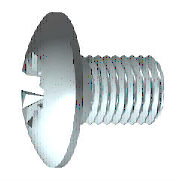
# Autodesk Inventor part: ANSI B18.6.3 - No. 2 - 56 - 5/8, CRTHMSTII(1)
Saved by Autodesk Inventor 2022.3 (Build 263350000, 350)
## iProperties
Created: 2021-02-01
Part Number: ANSI B18.6.3 - No. 2 - 56 - 5/8, CRTHMSTII(1)
Material: Steel, Mild
Description: Cross Recessed Truss Head Machine Screw - Type IA
Document SubType Name: Modeling
Standard: ANSI B18.6.3
Designer: Nathan Cai
Standard Revision: 2003
Standards Organization: ANSI
Language: en-US
Size Designation: No. 2 - 56 - 5/8
Categories: <MemberInstance><Categories><Category DisplayName="Fasteners" InternalName="e4da775c-781d-43d5-af7c-5136215cf5a6" Mnemonic="FSTN"><Category DisplayName="Bolts" InternalName="536e6df0-f778-49ac-b2f2-25c71d2aa0b2" Mnemonic="SCRW"><CategoryParameter DisplayName="Nominal Diameter Designation" InternalName="03caf894-eafd-4c09-a035-916ac084b87b" Mnemonic="nomdiadesig"/><CategoryParameter DisplayName="Nominal Length" InternalName="238ecbaf-3e6c-45dd-aa95-4068c8e0fd02" Mnemonic="nomlen"/><CategoryParameter DisplayName="Thread Designation" InternalName="586d5e89-370a-4089-914f-0110033585c7" Mnemonic="thrdesign"/><CategoryParameter DisplayName="Thread Series Designation" InternalName="87c5849c-b3a5-4c3e-9c9b-2feecef9be86" Mnemonic="thrserdsgn"/><CategoryParameter DisplayName="Nominal Diameter" InternalName="8bbe3f8e-44cf-40a9-a251-3a6edc8168d6" Mnemonic="nomdia"/><CategoryParameter DisplayName="Thread Type" InternalName="b4bbb7bc-d6aa-4c9f-a9a9-4152b9f6fe49" Mnemonic="thrtype"/><CategoryParameter DisplayName="Thread Pitch" InternalName="bb82302e-82d8-4176-8fc1-c5d7bb17d5ad" Mnemonic="pitch1"/><CategoryParameter DisplayName="Threads per Unit" InternalName="bdc6e7d2-ffd0-4d9c-a173-16b95ebb912d" Mnemonic="thrperunit1"/><CategoryParameter DisplayName="Thread Class" InternalName="ebc0d23b-2cc6-4d2a-b376-d52aae53bab6" Mnemonic="thrclss"/><Category DisplayName="Round Head" InternalName="df3578aa-538f-4805-96a8-2439eb0c3cf7" Mnemonic="RNDSCRW"><CategoryParameter DisplayName="Grip Length" InternalName="2c6ace26-543b-4217-91c4-9cdf8c3ec6f1" Mnemonic="grplen"/><CategoryParameter DisplayName="Head Height" InternalName="2d152238-84fe-49ae-94c3-3fee884c292b" Mnemonic="headh"/><CategoryParameter DisplayName="Property Class" InternalName="85496db6-1567-48ed-b0d4-aa1f03366005" Mnemonic="propclss"/><CategoryParameter DisplayName="Thread Length" InternalName="a1e5edc5-4ca7-4847-8786-65b14d35af16" Mnemonic="thrlen"/><CategoryParameter DisplayName="Shank Diameter" InternalName="c22f1a48-b8d5-43ef-ac5e-546ba91c0bd6" Mnemonic="grpdia"/><CategoryParameter DisplayName="Head Diameter" InternalName="e71ee7a1-06fd-425c-ba3b-09769885677c" Mnemonic="headdia"/></Category></Category></Category><Category DisplayName="DataType" InternalName="23b78d0f-2648-40c6-8793-ca6db495c9e8" Mnemonic="DATATYPE"><CategoryParameter DisplayName="DisplayName" InternalName="05415f3d-3907-474b-a020-eb9d644f4cf3" Mnemonic="DISPLAYNAME"/><CategoryParameter DisplayName="Standard" InternalName="0c0a119c-1e12-4c84-803f-101930972f5e" Mnemonic="STANDARD"/><CategoryParameter DisplayName="Description" InternalName="13903e3d-64b1-4950-80da-f627842ea37f" Mnemonic="DESCRIPTION"/><CategoryParameter DisplayName="Designation" InternalName="2675968c-4ce5-49e0-a4f5-552d29089031" Mnemonic="DESIGNATION"/><CategoryParameter DisplayName="Default Row" InternalName="2af9ec52-faaa-4026-b378-f9fa4afca842" Mnemonic="DEFAULTROW"/><CategoryParameter DisplayName="Folder Name" InternalName="3f06958e-8713-4116-9be7-ed6184ecc97b" Mnemonic="FOLDERNAME"/><CategoryParameter DisplayName="Revision Guid" InternalName="45a75005-10b1-4dfc-8d6d-dfe629f0b93c" Mnemonic="REVISIONGUID"/><CategoryParameter DisplayName="FileName" InternalName="8b46a4cc-9585-4fed-90c3-899f57e09a73" Mnemonic="FILENAME"/><CategoryParameter DisplayName="StdsOrg" InternalName="8f5914e1-4693-403f-8ab5-d37768198c9d" Mnemonic="STDSORG"/><CategoryParameter DisplayName="Family Version" InternalName="914462f6-6e19-4b14-ba84-155b9680b1d0" Mnemonic="FAMILYREVISION"/><CategoryParameter DisplayName="Standard Revision" InternalName="91d5a463-65c2-4fde-b823-3b7fea5e8e17" Mnemonic="STANDARDREVISION"/><CategoryParameter DisplayName="Member Revision" InternalName="a65d44b9-392f-4f4f-857b-e4b3d54996fe" Mnemonic="MEMBERREVISION"/><CategoryParameter DisplayName="ClipFormat" InternalName="bc51e27b-3422-4e78-93ef-cec197ddf230" Mnemonic="CLIPFORMAT"/><CategoryParameter DisplayName="Manufacturer" InternalName="cd6c7a72-a28a-4e50-99a9-2c7f4e13e5ad" Mnemonic="MANUFACTURER"/><CategoryParameter DisplayName="InternalName" InternalName="cf1d0246-76d9-4b4a-8305-fa0409afb5c1" Mnemonic="INTERNALNAME"/><CategoryParameter DisplayName="IsMetric" InternalName="e2385c5b-1ea4-4823-96a8-8de651266ec3" Mnemonic="ISMETRIC"/><Category DisplayName="Part" InternalName="c0e0b642-3bcb-4cc8-9e80-f96d35c4afa4" Mnemonic="PART"><CategoryParameter DisplayName="Part Number" InternalName="016b6077-bfbe-49bd-92c9-d8d59c39c941" Mnemonic="PARTNUMBER"/><CategoryParameter DisplayName="Stock Number" InternalName="4dba7c1c-e26c-444e-836c-b08b433409a8" Mnemonic="STOCKNUMBER"/><CategoryParameter DisplayName="Material Key" InternalName="5c9a8adb-dd2b-4535-b97f-0a94a95fe41f" Mnemonic="MATERIALKEY"/><CategoryParameter DisplayName="Material" InternalName="818a152a-d3c3-49ca-80ee-df7d91421b8e" Mnemonic="MATERIAL"/></Category></Category><Category DisplayName="Legacy Map DA" InternalName="924fff40-ddd0-4eff-ad42-30e3774ef79e" Mnemonic="LEGACYMAPDA"><CategoryParameter DisplayName="DACookie" InternalName="316934ee-8fe1-4c7a-9c36-f2d79e1add1a" Mnemonic="DACOOKIE"/></Category><Category DisplayName="LegacyMap" InternalName="cd87c42b-3e48-431e-b5c0-1cbeb14dfe77" Mnemonic="LEGACYMAP"><CategoryParameter DisplayName="unique DA member ID" InternalName="0918ad47-427f-4fed-ae26-24c81c58f590" Mnemonic="DACOOKIE"/><CategoryParameter DisplayName="Merge11 ID" InternalName="0ee8fb18-e2ed-4f39-96f6-1f4b5f50aa71" Mnemonic="MERGE11"/><CategoryParameter DisplayName="unique CC member ID" InternalName="5193edd4-b2b0-4ab4-9d54-de900eee34e0" Mnemonic="CCCOOKIE"/><CategoryParameter DisplayName="Split ID" InternalName="72b5c83c-be7f-45c4-ae51-9160ea6deb26" Mnemonic="SPLIT"/><CategoryParameter DisplayName="MemberID" InternalName="8e5e0294-fc51-4c8f-b3d7-003dc5ed94f6" Mnemonic="MEMBERID"/><CategoryParameter DisplayName="CatalogName" InternalName="d99d1e27-aa94-4de2-af4c-c348882a6f4f" Mnemonic="CATALOGNAME"/><CategoryParameter DisplayName="FamilyNumber" InternalName="e705e1f4-09cb-413e-91f9-551b4188271e" Mnemonic="FAMILYNUMBER"/></Category></Categories><FamilyTemplate Id="sa0019"><FamilyTemplateParameters><FamilyTemplateParameter ObjectType="kUserParameterObject" ValueType="xs:double" Id="1" ObjectReferenceKey="GUL"/><FamilyTemplateParameter ObjectType="kUserParameterObject" ValueType="xs:double" Id="2" ObjectReferenceKey="SPD"/><FamilyTemplateParameter ObjectType="kUserParameterObject" ValueType="xs:double" Id="3" ObjectReferenceKey="KOD"/><FamilyTemplateParameter ObjectType="kUserParameterObject" ValueType="xs:double" Id="4" ObjectReferenceKey="SBR"/><FamilyTemplateParameter ObjectType="kUserParameterObject" ValueType="xs:double" Id="5" ObjectReferenceKey="KR"/><FamilyTemplateParameter ObjectType="kUserParameterObject" ValueType="xs:double" Id="6" ObjectReferenceKey="PTC"/><FamilyTemplateParameter ObjectType="kUserParameterObject" ValueType="xs:double" Id="7" ObjectReferenceKey="SDM"/><FamilyTemplateParameter ObjectType="kUserParameterObject" ValueType="xs:double" Id="8" ObjectReferenceKey="THREADDIA"/><FamilyTemplateParameter ObjectType="kUserParameterObject" ValueType="xs:double" Id="9" ObjectReferenceKey="GEL"/><FamilyTemplateParameter ObjectType="kUserParameterObject" ValueType="xs:double" Id="10" ObjectReferenceKey="TOA"/><FamilyTemplateParameter ObjectType="kUserParameterObject" ValueType="xs:double" Id="11" ObjectReferenceKey="BDM"/><FamilyTemplateParameter ObjectType="kUserParameterObject" ValueType="xs:double" Id="12" ObjectReferenceKey="NLG"/><FamilyTemplateParameter ObjectType="kUserParameterObject" ValueType="xs:double" Id="13" ObjectReferenceKey="STI"/><FamilyTemplateParameter ObjectType="kUserParameterObject" ValueType="xs:double" Id="14" ObjectReferenceKey="TPU"/><FamilyTemplateParameter ObjectType="kUserParameterObject" ValueType="xs:double" Id="15" ObjectReferenceKey="KOH"/><FamilyTemplateParameter ObjectType="kUserParameterObject" ValueType="xs:double" Id="16" ObjectReferenceKey="NND"/><FamilyTemplateParameter ObjectType="kUserParameterObject" ValueType="xs:double" Id="17" ObjectReferenceKey="GD"/><FamilyTemplateParameter ObjectType="kUserParameterObject" ValueType="xs:double" Id="18" ObjectReferenceKey="GAL"/><FamilyTemplateParameter ObjectType="kUserParameterObject" ValueType="xs:double" Id="19" ObjectReferenceKey="GD1"/><FamilyTemplateParameter ObjectType="kUserParameterObject" ValueType="xs:double" Id="116" ObjectReferenceKey="RR"/><FamilyTemplateParameter ObjectType="kPropertyObject" ValueType="xs:string" Id="100" ObjectReferenceKey="{32853F0F-3444-11d1-9E93-0060B03C1CA6}" SubObjectId="52"/><FamilyTemplateParameter ObjectType="kPropertyObject" ValueType="xs:string" Id="105" ObjectReferenceKey="{32853F0F-3444-11d1-9E93-0060B03C1CA6}" SubObjectId="5"/><FamilyTemplateParameter ObjectType="kPartComponentDefinitionObject" ValueType="xs:string" Id="110" SubObjectId="Material"/><FamilyTemplateParameter ObjectType="kThreadFeatureObject" ValueType="xs:structure" Id="300" ObjectReferenceKey="1002000010000000aa0f0000000000008000000000000000" SubObjectId="ThreadInfo"><FamilyTemplateParameter ObjectType="" ValueType="xs:string" Id="301" SubObjectId="ThreadDesignation"/><FamilyTemplateParameter ObjectType="" ValueType="xs:string" Id="302" SubObjectId="ThreadType"/><FamilyTemplateParameter ObjectType="" ValueType="xs:string" Id="303" SubObjectId="ThreadClass"/></FamilyTemplateParameter></FamilyTemplateParameters></FamilyTemplate><CategoryParameterMap><ParamToTemplateMap><ParamToTemplate CategoryParameter="//CategoryParameter[@InternalName='05415f3d-3907-474b-a020-eb9d644f4cf3']" ConstantValue="Cross Recessed Truss Head Machine Screw - Type IA - Inch"/><ParamToTemplate CategoryParameter="//CategoryParameter[@InternalName='cf1d0246-76d9-4b4a-8305-fa0409afb5c1']" ConstantValue="e32b86c7-b789-4434-bfba-ffda7e126eb0"/><ParamToTemplate CategoryParameter="//CategoryParameter[@InternalName='3f06958e-8713-4116-9be7-ed6184ecc97b']" ConstantValue="ANSI B18.6.3(28)"/><ParamToTemplate CategoryParameter="//CategoryParameter[@InternalName='914462f6-6e19-4b14-ba84-155b9680b1d0']" ConstantValue="10"/><ParamToTemplate CategoryParameter="//CategoryParameter[@InternalName='bc51e27b-3422-4e78-93ef-cec197ddf230']" ConstantValue="CF_INVENTOR.STDPARTS"/><ParamToTemplate CategoryParameter="//CategoryParameter[@InternalName='e2385c5b-1ea4-4823-96a8-8de651266ec3']" ConstantValue="false"/><ParamToTemplate CategoryParameter="//CategoryParameter[@InternalName='13903e3d-64b1-4950-80da-f627842ea37f']" ConstantValue="Cross Recessed Truss Head Machine Screw - Type IA"/><ParamToTemplate CategoryParameter="//CategoryParameter[@InternalName='8f5914e1-4693-403f-8ab5-d37768198c9d']" ConstantValue="ANSI"/><ParamToTemplate CategoryParameter="//CategoryParameter[@InternalName='0c0a119c-1e12-4c84-803f-101930972f5e']" ConstantValue="ANSI B18.6.3"/><ParamToTemplate CategoryParameter="//CategoryParameter[@InternalName='cd6c7a72-a28a-4e50-99a9-2c7f4e13e5ad']" TemplateParameter="104"/><ParamToTemplate CategoryParameter="//CategoryParameter[@InternalName='91d5a463-65c2-4fde-b823-3b7fea5e8e17']" ConstantValue="2003"/><ParamToTemplate CategoryParameter="//CategoryParameter[@InternalName='45a75005-10b1-4dfc-8d6d-dfe629f0b93c']" ConstantValue="33de6b0a-c454-4489-82c3-c7e6c35f5d89"/><ParamToTemplate CategoryParameter="//CategoryParameter[@InternalName='2af9ec52-faaa-4026-b378-f9fa4afca842']" ConstantValue="10"/><ParamToTemplate CategoryParameter="//CategoryParameter[@InternalName='d99d1e27-aa94-4de2-af4c-c348882a6f4f']" ConstantValue="ANSI"/><ParamToTemplate CategoryParameter="//CategoryParameter[@InternalName='8b46a4cc-9585-4fed-90c3-899f57e09a73']" ConstantValue="ANSI B18.6.3 - 2-56 UNC - 0.625(12)"/><ParamToTemplate CategoryParameter="//CategoryParameter[@InternalName='a65d44b9-392f-4f4f-857b-e4b3d54996fe']" ConstantValue="ABF65F4B-D9A5-4458-8652-3F63C1D7C885"/><ParamToTemplate CategoryParameter="//CategoryParameter[@InternalName='2c6ace26-543b-4217-91c4-9cdf8c3ec6f1']" ConstantValue="0.04464"/><ParamToTemplate CategoryParameter="//CategoryParameter[@InternalName='ebc0d23b-2cc6-4d2a-b376-d52aae53bab6']" ConstantValue="2A"/><ParamToTemplate CategoryParameter="//CategoryParameter[@InternalName='87c5849c-b3a5-4c3e-9c9b-2feecef9be86']" ConstantValue="UNC"/><ParamToTemplate CategoryParameter="//CategoryParameter[@InternalName='03caf894-eafd-4c09-a035-916ac084b87b']" ConstantValue="#2"/><ParamToTemplate CategoryParameter="//CategoryParameter[@InternalName='b4bbb7bc-d6aa-4c9f-a9a9-4152b9f6fe49']" ConstantValue="ANSI Unified Screw Threads"/><ParamToTemplate CategoryParameter="//CategoryParameter[@InternalName='e705e1f4-09cb-413e-91f9-551b4188271e']" ConstantValue="133"/><ParamToTemplate CategoryParameter="//CategoryParameter[@InternalName='8e5e0294-fc51-4c8f-b3d7-003dc5ed94f6']" ConstantValue="130"/><ParamToTemplate CategoryParameter="//CategoryParameter[@InternalName='316934ee-8fe1-4c7a-9c36-f2d79e1add1a']" ConstantValue="*Ans~A1863E2~2-56x0.625~0.625~UNC*"/><ParamToTemplate CategoryParameter="//CategoryParameter[@InternalName='2675968c-4ce5-49e0-a4f5-552d29089031']" TemplateParameter="100"/><ParamToTemplate CategoryParameter="//CategoryParameter[@InternalName='c22f1a48-b8d5-43ef-ac5e-546ba91c0bd6']" TemplateParameter="17"/><ParamToTemplate CategoryParameter="//CategoryParameter[@InternalName='a1e5edc5-4ca7-4847-8786-65b14d35af16']" TemplateParameter="9"/><ParamToTemplate CategoryParameter="//CategoryParameter[@InternalName='e71ee7a1-06fd-425c-ba3b-09769885677c']" TemplateParameter="3"/><ParamToTemplate CategoryParameter="//CategoryParameter[@InternalName='2d152238-84fe-49ae-94c3-3fee884c292b']" TemplateParameter="15"/><ParamToTemplate CategoryParameter="//CategoryParameter[@InternalName='818a152a-d3c3-49ca-80ee-df7d91421b8e']" TemplateParameter="110"/><ParamToTemplate CategoryParameter="//CategoryParameter[@InternalName='238ecbaf-3e6c-45dd-aa95-4068c8e0fd02']" TemplateParameter="12"/><ParamToTemplate CategoryParameter="//CategoryParameter[@InternalName='8bbe3f8e-44cf-40a9-a251-3a6edc8168d6']" TemplateParameter="16"/><ParamToTemplate CategoryParameter="//CategoryParameter[@InternalName='016b6077-bfbe-49bd-92c9-d8d59c39c941']" TemplateParameter="105"/><ParamToTemplate CategoryParameter="//CategoryParameter[@InternalName='bb82302e-82d8-4176-8fc1-c5d7bb17d5ad']" TemplateParameter="6"/><ParamToTemplate CategoryParameter="//CategoryParameter[@InternalName='586d5e89-370a-4089-914f-0110033585c7']" TemplateParameter="301"/><ParamToTemplate CategoryParameter="//CategoryParameter[@InternalName='bdc6e7d2-ffd0-4d9c-a173-16b95ebb912d']" TemplateParameter="14"/></ParamToTemplateMap></CategoryParameterMap></MemberInstance>
Density: 7.85 g/cm^3
Appearance: Semi-Polished
IsCustomPart: 0
Author: Nathan Cai
Autodesk Inventor part; units mm, degrees
ref_plane "YZ Plane" through (0, 0, 0) normal (1, 0, 0) x (0, 1, 0)
sketch "Sketch1" plane through (0, 0, 0) normal (0, 0, 1) x (1, 0, 0)
  line L0 (15.875, 0) -> (15.875, 1.0922)
  line L1 (15.875, 1.0922) -> (0, 1.0922)
  line L2 (3.9624, 5.08) -> (3.9624, 5.08)
  arc A0 (-0.2296, 2.4638) -> (-1.3462, 0) centre (1.9304, 0) ccw
  line L3 (-1.3462, 0) -> (-1.3462, 2.4638)
  line L4 (-1.1677, 1.0667) -> (-0.4197, 0.6938)
  line L5 (-0.4197, 0.6938) -> (-0.0508, 0)
  line L6 (-0.0508, 0) -> (15.875, 0)
  line L7 (-5.1098, 0) -> (19.3725, 0) projected
  line L8 (0, -1.016) -> (0, 6.096) projected
  line L9 (-1.1677, 1.0667) -> (-1.3462, 1.1557) construction
  line L10 (-0.2296, 2.4638) -> (-1.3462, 2.4638)
  line L11 (-0.2296, 2.4638) -> (0, 2.4638)
  line L12 (0, 2.4638) -> (0, 1.0922)
  dimension "d1" = 2.1844
  dimension "d2" = 1.2954
  dimension "d16" = 2.3114
  dimension "d17" = 62
  dimension "d19" = 26.5
  dimension "d23" = 4.9276
  dimension "d25" = 1.3462
  dimension "d26" = 3.2766
  dimension "d28" = 15.875
  constraints: 22 end point, 4 collinear, 4 point on circle, 3 point on line, 2 parallel, 2 perpendicular, 1 centre point, 1 horizontal, 1 tangent
  measures "d1" diameter of L1 L6
  measures "d2" distance from line of L5.end L3
  measures "d16" diameter of L9.end L6
  measures "d17" angle of L5 L6
  measures "d19" angle of L4 L6
  measures "d23" diameter of L11.end L6
  measures "d25" distance between parallel lines of L3 L12
  measures "d26" radius of A0
  measures "d28" distance between parallel lines of L0 L12
revolve "Body" add sketch "Sketch1" angle 360 about axis through (-0.0508, 0, 0) along (1, 0, 0) contours L6 L8 L1 L0 | L6 L5 L4 A0 L11 L8
ref_plane "IDS_WORKPLANE{1}" through (-1.3462, 0, 0) normal (1, 0, 0) x (0, 1, 0)
sketch "Sketch2" plane through (-1.3462, 0, 0) normal (1, 0, 0) x (0, 1, 0)
  circle A0 centre (0, 0) radius 2.4638 projected
  line L0 (-4.3007, 0) -> (8.5575, 0) projected
  line L1 (0, -4.3007) -> (0, 8.5575) projected
  line L2 (0, 1.1557) -> (0, 0) construction
  line L3 (0, 0) -> (1.1557, 0) construction
  arc A1 (0.4623, 0) -> (0, 0.4623) centre (0, 0) ccw construction
  line L4 (0, 0) -> (6.7207, 6.7207) construction
  line L5 (0.3683, 1.0954) -> (0.1895, 0.5459)
  line L6 (1.0954, 0.3683) -> (0.5459, 0.1895)
  arc A2 (0.1895, 0.5459) -> (0.4104, 0.4104) centre (0.3162, 0.5047) ccw
  arc A3 (0.4104, 0.4104) -> (0.5459, 0.1895) centre (0.5047, 0.3162) ccw
  arc A4 (1.1557, 0) -> (1.0954, 0.3683) centre (0, 0) ccw
  arc A5 (0.3683, 1.0954) -> (0, 1.1557) centre (0, 0) ccw
  arc A6 (1.0954, 0.3683) -> (0.3683, 1.0954) centre (0, 0) ccw
  line L7 (0.3683, -1.0954) -> (0.1895, -0.5459)
  line L8 (1.0954, -0.3683) -> (0.5459, -0.1895)
  arc A7 (0.4104, -0.4104) -> (0.1895, -0.5459) centre (0.3162, -0.5047) ccw
  arc A8 (0.5459, -0.1895) -> (0.4104, -0.4104) centre (0.5047, -0.3162) ccw
  arc A9 (1.0954, -0.3683) -> (1.1557, 0) centre (0, 0) ccw
  arc A10 (0, -1.1557) -> (0.3683, -1.0954) centre (0, 0) ccw
  arc A11 (0.3683, -1.0954) -> (1.0954, -0.3683) centre (0, 0) ccw
  line L9 (-0.3683, 1.0954) -> (-0.1895, 0.5459)
  line L10 (-1.0954, 0.3683) -> (-0.5459, 0.1895)
  arc A12 (-0.4104, 0.4104) -> (-0.1895, 0.5459) centre (-0.3162, 0.5047) ccw
  arc A13 (-0.5459, 0.1895) -> (-0.4104, 0.4104) centre (-0.5047, 0.3162) ccw
  arc A14 (-1.0954, 0.3683) -> (-1.1557, 0) centre (0, 0) ccw
  arc A15 (0, 1.1557) -> (-0.3683, 1.0954) centre (0, 0) ccw
  arc A16 (-0.3683, 1.0954) -> (-1.0954, 0.3683) centre (0, 0) ccw
  arc A17 (-0.3683, -1.0954) -> (0, -1.1557) centre (0, 0) ccw
  arc A18 (-1.0954, -0.3683) -> (-0.3683, -1.0954) centre (0, 0) ccw
  arc A19 (-1.1557, 0) -> (-1.0954, -0.3683) centre (0, 0) ccw
  line L11 (-1.0954, -0.3683) -> (-0.5459, -0.1895)
  line L12 (-0.3683, -1.0954) -> (-0.1895, -0.5459)
  arc A20 (-0.1895, -0.5459) -> (-0.4104, -0.4104) centre (-0.3162, -0.5047) ccw
  arc A21 (-0.4104, -0.4104) -> (-0.5459, -0.1895) centre (-0.5047, -0.3162) ccw
  arc A22 (0.5778, 0) -> (0, 0.5778) centre (0, 0) ccw construction
  dimension "d4" = 45
  dimension "d5" = 0.9246
  dimension "d6" = 2.3114
  dimension "d7" = 0.3683
  dimension "d20" = 1.1557
  constraints: 46 point on circle, 25 symmetric about line, 22 centre point, 22 end point, 6 tangent, 4 coincident, 3 collinear, 3 point on line, 1 midpoint, 1 perpendicular, 22 other
  measures "d4" angle of L4 L3
  measures "d5" diameter of A1
  measures "d6" diameter of A6
  measures "d7" distance from line of L5.start L2
  measures "d20" diameter of A22
extrude "Slot" add sketch "Sketch2" along normal up to next contours L6 A3 A2 L5 A6 | A11 L7 A7 A8 L8 | L9 A12 A13 L10 A16 | A18 L11 A21 A20 L12
revolve "Cut" cut sketch "Sketch1" angle 360 about axis through (-10, 0, 0) along (1, 0, 0) contours L3 L10 A0
sketch "Sketch4" plane through (-1.3462, 0, 0) normal (1, 0, 0) x (0, 1, 0)
  circle A0 centre (0, 0) radius 2.4638 projected
  line L0 (-8.9998, 0) -> (8.9998, 0) projected
  line L1 (0, -8.9998) -> (0, 8.9998) projected
  line L2 (0, 0) -> (6.4284, 6.4284) construction
  circle A1 centre (0, 0) radius 0.1842 construction
  line L3 (0, 0) -> (6.4284, -6.4284) construction
  line L4 (0, 0) -> (-6.4284, 6.4284) construction
  line L5 (0, 0) -> (-6.4284, -6.4284) construction
  line L6 (0.8172, 0.8172) -> (0, 0.1842)
  line L7 (-0.8172, 0.8172) -> (-0.1842, 0)
  line L8 (-0.8172, -0.8172) -> (0, -0.1842)
  line L9 (0.8172, -0.8172) -> (0.1841, 0)
  line L10 (0.8172, 0.8172) -> (0.1841, 0)
  line L11 (-0.8172, 0.8172) -> (0, 0.1842)
  line L12 (-0.8172, -0.8172) -> (-0.1842, 0)
  line L13 (0.8172, -0.8172) -> (0, -0.1842)
  circle A2 centre (0, 0) radius 1.1557 construction
  dimension "d11" = 0.3683
  dimension "d14" = 45
  dimension "d29" = 0.8172
  constraints: 25 end point, 7 point on circle, 7 point on line, 3 symmetric about line, 2 centre point, 2 coincident, 2 perpendicular, 3 other
  measures "d11" diameter of A1
  measures "d14" angle of L2 L0
  measures "d29" distance from line of L0 L6.start
extrude "Star Cut" cut sketch "Sketch4" along normal blind 1.3462 draft -30 contours L9 L13 L1 L0 | L0 L1 L6 L10 | L1 L0 L7 L11 | L8 L12 L0 L1
fillet "Fillet1" radius 0.1473 5 edges at (-1.1677, 0, 1.0667) (-1.1677, -1.0667, 0) (-1.1677, 0, -1.0667) (-1.1677, 1.0526, -0.1727) (-1.1677, 1.0526, 0.1727)
thread "Thread" size "2-56 UNC" class "2A" standard "ANSI Unified Screw Threads" length 14.7411
chamfer "Chamfer" distance 0.2268 angle 45 1 edges at (15.875, -1.0922, 0)
ref_plane "Work Plane3" through (2.3813, 0, 0) normal (0, 1, 0) x (1, 0, 0)
equation "\"d11\" = 0.5 * SBR"
equation "\"d29\" = 0.353553 * SDM"
equation "\"d12\" = KOH"
equation "\"d5\" = 0.4 * SDM"
equation "\"d6\" = SDM"
equation "\"d7\" = 0.5 * SBR"
equation "\"d20\" = 0.5 * SDM"
equation "\"d1\" = GD"
equation "\"d2\" = STI"
equation "\"d16\" = SDM"
equation "\"d23\" = KOD"
equation "\"d25\" = KOH"
equation "\"d26\" = KR"
equation "\"d28\" = NLG"
equation "\"d22\" = 0.2 * SBR"
equation "\"d8\" = GEL"
equation "\"d78\" = 0.5 * RR"
equation "\"GD\" = NND"
equation "\"NLG\" = 15.875"
equation "\"GEL\" = 14.74114"
equation "\"KOD\" = 4.9276"
equation "\"KOH\" = 1.3462"
equation "\"SDM\" = 2.3114"
equation "\"STI\" = 1.2954"
equation "\"SBR\" = 0.7366"
equation "\"d3\" = -KOH"
equation "\"KR\" = 3.2766"
equation "\"GUL\" = 0"
equation "\"SPD\" = 1.35357"
equation "\"THREADDIA\" = 2.1844"
equation "\"TOA\" = 30deg"
equation "\"BDM\" = NND"
equation "\"NND\" = 2.1844"
equation "\"GAL\" = 0.45466"
equation "\"GD1\" = 1.62814"
equation "\"RR\" = 0.453571"
body "Solid1"
